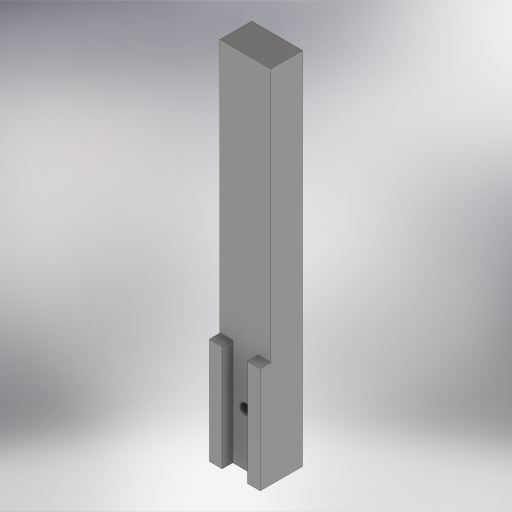
# Autodesk Inventor part: Braço1
Saved by Autodesk Inventor 2023 (Build 270158000, 158)
## iProperties
Created: 2023-03-17
Part Number: Braço1
Material: Aço inoxidável
Document SubType Name: Sheet Metal
Designer: Mateus
Mass: 254.4 g
Surface Area: 73.6 cm^2
Volume: 31.8 cm^3
Density: 8 g/cm^3
Sheet Metal Rule: Padrão_mm
Appearance: Semipolido
Author: Mateus
Autodesk Inventor part; units mm, degrees
ref_plane "YZ Plane" through (0, 0, 0) normal (1, 0, 0) x (0, 1, 0)
ref_plane "XZ Plane" through (0, 0, 0) normal (0, 1, 0) x (-1, 0, 0)
ref_plane "XY Plane" through (0, 0, 0) normal (0, 0, 1) x (1, 0, 0)
sketch "Esboço1" plane through (0, 0, 0) normal (0, 1, 0) x (-1, 0, 0)
  line L0 (0, 0) -> (24, 0)
  line L1 (24, 0) -> (24, -15)
  line L2 (24, -15) -> (0, -15)
  line L3 (0, -15) -> (0, 0)
  dimension "d0" = 24
  dimension "d1" = 15
  constraints: 8 end point, 2 parallel, 1 horizontal, 1 perpendicular
  measures "d0" distance of L1.end L2.end
  measures "d1" distance of L0.end L1.end
extrude "Extrusão1" add sketch "Esboço1" along normal blind 170
sketch "Esboço2" plane through (-24, 0, 0) normal (0, 0, 1) x (1, 0, 0)
  line L0 (24, 0) -> (0, 0) projected
  line L1 (0, 0) -> (6, 0)
  line L2 (6, 0) -> (6, 50)
  line L3 (6, 50) -> (0, 50)
  line L4 (0, 50) -> (0, 0)
  line L5 (24, 0) -> (18, 0)
  line L6 (18, 0) -> (18, 50)
  line L7 (18, 50) -> (24, 50)
  line L8 (24, 50) -> (24, 0)
  dimension "d4" = 12
  dimension "d5" = 50
  constraints: 16 end point, 4 parallel, 2 horizontal, 2 perpendicular, 1 collinear, 1 point on line
  measures "d4" distance between parallel lines of L2 L6
  measures "d5" distance of L7.end L0.start
extrude "Extrusão2" add sketch "Esboço2" along normal blind 5
sketch "Esboço3" plane through (0, 0, -15) normal (0, 0, -1) x (-1, 0, 0)
  line L0 (0, 0) -> (24, 0) projected
  line L1 (0, 0) -> (0, 170) projected
  point P0 (12, 25)
  dimension "d8" = 24
  dimension "d9" = 12
  dimension "d10" = 25
  measures "d8" distance of L0.start L0.end
  measures "d9" distance from line of L1 point (12, 25)
  measures "d10" distance from line of L0 point (12, 25)
hole "Furo1" at (-12, 25, -15) direction (0, 0, 1) diameter 4.917 depth 15 tip angle 118 thread size "M6x1" class "6H" standard "ISO Metric profile"
equation "\"d9\" = 0.5 * d8"
equation "\"d16\" = Espessura"
equation "\"Raio_vergadura\" = Espessura"
equation "\"Largura_alívio_de_vergadura\" = Espessura"
equation "\"Profundidade_alívio_de_vergadura\" = 0.5 * Espessura"
equation "\"Tamanho_alívio_de_dobra\" = 4 * Espessura"
equation "\"Remanescente_mínimo\" = 2 * Espessura"
equation "\"Raiodetransição\" = Raio_vergadura"
equation "\"Tamanho_de_raio_de_Jacobi\" = Raio_vergadura"
equation "\"TamanhoFolga\" = Espessura"
equation "\"Espessura\" = 0.5"
